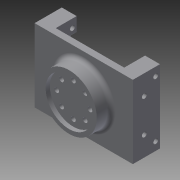
# Autodesk Inventor part: 90turnmount
Saved by Autodesk Inventor 2015 (Build 190159000, 159)
## iProperties
Created: 2016-12-16
Part Number: 90turnmount
Material: Generic
Document SubType Name: Modeling
Designer: Rudge-Top
Density: 1 g/cm^3
Appearance: Default
Author: Rudge-Top
Autodesk Inventor part; units mm, degrees
ref_plane "YZ Plane" through (0, 0, 0) normal (1, 0, 0) x (0, 1, 0)
ref_plane "XZ Plane" through (0, 0, 0) normal (0, 1, 0) x (-1, 0, 0)
ref_plane "XY Plane" through (0, 0, 0) normal (0, 0, 1) x (1, 0, 0)
sketch "Sketch1" plane through (0, 0, 0) normal (0, 1, 0) x (-1, 0, 0)
  circle A0 centre (0, 0) radius 11.25
  circle A1 centre (0, 0) radius 13.25
  dimension "d0" = 22.5
  dimension "d1" = 26.5
  constraints: 2 centre point, 2 coincident
  measures "d0" diameter of A0
  measures "d1" diameter of A1
extrude "Extrusion1" add sketch "Sketch1" along normal blind 2
sketch "Sketch2" plane through (0, 2, 0) normal (0, 1, 0) x (1, 0, 0)
  circle A0 centre (0, 0) radius 11.25 projected
  circle A1 centre (0, 0) radius 13.25 projected
extrude "Extrusion2" add sketch "Sketch2" along normal blind 5 contours A0 | A1
sketch "Sketch3" plane through (0, 7, 0) normal (0, 1, 0) x (1, 0, 0)
  line L0 (23.55, -17.5) -> (-23.55, -17.5)
  line L1 (-23.55, -17.5) -> (-23.55, 17.5)
  line L2 (-23.55, 17.5) -> (23.55, 17.5)
  line L3 (23.55, 17.5) -> (23.55, -17.5)
  point P0 (0, 0)
  dimension "d6" = 47.1
  dimension "d7" = 35
  dimension "d8" = 17.5
  dimension "d9" = 23.55
  constraints: 8 end point, 2 parallel, 1 horizontal, 1 perpendicular
  measures "d6" distance of L1.end L2.end
  measures "d7" distance of L2.end L0.start
  measures "d8" distance from line of L0 point (0, 0)
  measures "d9" distance from line of point (0, 0) L3
extrude "Extrusion3" add sketch "Sketch3" along normal blind 3
fillet "Fillet1" radius 2 1 edges at (-13.25, 7, 0)
sketch "Sketch4" plane through (0, 10, 0) normal (0, 1, 0) x (1, 0, 0)
  line L0 (-23.55, 17.5) -> (23.55, 17.5) projected
  line L1 (23.55, -17.5) -> (16.4, -17.5)
  line L2 (16.4, -17.5) -> (16.4, 17.5)
  line L3 (16.4, 17.5) -> (23.55, 17.5)
  line L4 (23.55, 17.5) -> (23.55, -17.5)
  line L5 (-23.55, -17.5) -> (-16.4, -17.5)
  line L6 (-16.4, -17.5) -> (-16.4, 17.5)
  line L7 (-16.4, 17.5) -> (-23.55, 17.5)
  line L8 (-23.55, 17.5) -> (-23.55, -17.5)
  point P0 (0, 0)
  dimension "d13" = 7.15
  dimension "d14" = 7.15
  constraints: 16 end point, 4 parallel, 2 horizontal, 2 perpendicular, 2 point on line
  measures "d13" distance of L2.end L3.end
  measures "d14" distance of L7.end L6.end
extrude "Extrusion4" add sketch "Sketch4" along normal blind 10
sketch "Sketch5" plane through (23.55, 7, 17.5) normal (1, 0, 0) x (0, 0, -1)
  line L0 (35, 0) -> (0, 0) projected
  line L1 (35, 0) -> (35, 13) projected
  line L2 (0, 13) -> (35, 13) projected
  line L3 (0, 0) -> (0, 13) projected
  line L4 (35, 13) -> (0, 13) projected
  line L5 (17.5, 13) -> (17.5, 7.9729)
  point P0 (17.5, -7)
  point P1 (25.5, 5.5)
  point P2 (31, 11)
  point P3 (9.5, 5.5)
  point P4 (4, 11)
  dimension "d17" = 5.5
  dimension "d18" = 5.5
  dimension "d19" = 8
  dimension "d20" = 13.5
  constraints: 2 end point, 2 symmetric about line, 1 midpoint, 1 vertical
  measures "d17" distance from line of L0 point (25.5, 5.5)
  measures "d18" horizontal distance of point (31, 11) point (25.5, 5.5)
  measures "d19" distance from line of L5 point (25.5, 5.5)
  measures "d20" distance from line of L5 point (31, 11)
hole "Hole1" at (23.55, 12.5, -8) at (23.55, 18, -13.5) at (23.55, 18, 13.5) at (23.55, 12.5, 8) direction (-1, 0, 0) diameter 2.3 end through all
sketch "Sketch6" plane through (0, 20, 0) normal (0, 1, 0) x (1, 0, 0)
  line L0 (23.55, -17.5) -> (23.55, 17.5) projected
  line L1 (23.55, 17.5) -> (16.4, 17.5) projected
  line L2 (16.4, 17.5) -> (16.4, -17.5) projected
  line L3 (16.4, -17.5) -> (23.55, -17.5) projected
  line L4 (16.4, 17.5) -> (16.4, -17.5) projected
  line L5 (16.4, -10.5) -> (19.3, -10.5)
  line L6 (19.3, -10.5) -> (19.3, 10.5)
  line L7 (19.3, 10.5) -> (16.4, 10.5)
  line L8 (16.4, 10.5) -> (16.4, -10.5)
  point P0 (0, 0)
  dimension "d28" = 2.9
  dimension "d29" = 21
  dimension "d30" = 7
  constraints: 8 end point, 2 parallel, 1 horizontal, 1 perpendicular, 1 point on line
  measures "d28" distance of L7.end L6.end
  measures "d29" distance of L6.end L5.end
  measures "d30" distance between parallel lines of L5 L3
extrude "Extrusion5" cut sketch "Sketch6" against normal blind 5.1 contours L2 L7 L6 L5
sketch "Sketch7" plane through (0, 20, 0) normal (0, 1, 0) x (1, 0, 0)
  line L0 (-16.4, 17.5) -> (-23.55, 17.5) projected
  line L1 (-23.55, 17.5) -> (-23.55, -17.5) projected
  line L2 (-23.55, -17.5) -> (-16.4, -17.5) projected
  line L3 (-16.4, -17.5) -> (-16.4, 17.5) projected
  line L4 (-16.4, -10.6) -> (-19.3, -10.6)
  line L5 (-19.3, -10.6) -> (-19.3, -3.6)
  line L6 (-19.3, -3.6) -> (-16.4, -3.6)
  line L7 (-16.4, -3.6) -> (-16.4, -10.6)
  line L8 (-16.4, 10.6) -> (-19.3, 10.6)
  line L9 (-19.3, 10.6) -> (-19.3, 3.6)
  line L10 (-19.3, 3.6) -> (-16.4, 3.6)
  line L11 (-16.4, 3.6) -> (-16.4, 10.6)
  point P0 (0, 0)
  dimension "d33" = 2.9
  dimension "d34" = 7
  dimension "d35" = 6.9
  dimension "d36" = 2.9
  dimension "d37" = 7
  dimension "d38" = 6.9
  constraints: 16 end point, 4 parallel, 2 horizontal, 2 perpendicular, 2 point on line
  measures "d33" distance of L5.end L6.end
  measures "d34" distance of L4.end L5.end
  measures "d35" distance between parallel lines of L2 L4
  measures "d36" distance of L10.end L9.end
  measures "d37" distance of L9.end L8.end
  measures "d38" distance between parallel lines of L0 L8
extrude "Extrusion6" cut sketch "Sketch7" against normal blind 5.1 contours L3 L10 L9 L8 | L3 L4 L5 L6
fillet "Fillet2" radius 0.5 9 edges at (-16.4, 17.45, 10.6) (-16.4, 14.9, 7.1) (-16.4, 17.45, 3.6) (-16.4, 14.9, -7.1) (-16.4, 17.45, -3.6) (-16.4, 17.45, -10.6) (16.4, 17.45, 10.5) (16.4, 14.9, 0) (16.4, 17.45, -10.5)
sketch "Sketch8" plane through (0, 2, 0) normal (0, -1, 0) x (1, 0, 0)
  point P0 (0, 0)
  point P1 (0, -8)
  point P2 (5.6569, -5.6569)
  point P3 (8, 0)
  point P4 (5.6569, 5.6569)
  point P5 (0, 8)
  point P6 (-5.6569, 5.6569)
  point P7 (-8, 0)
  point P8 (-5.6569, -5.6569)
  dimension "d42" = 8
  dimension "d45" = 360
  constraints: 9 other
  measures "d42" distance of point (0, 0) point (0, -8)
hole "Hole2" at (0, 2, -8) at (5.6569, 2, -5.6569) at (8, 2, 0) at (5.6569, 2, 5.6569) at (0, 2, 8) at (-5.6569, 2, 5.6569) at (-8, 2, 0) at (-5.6569, 2, -5.6569) direction (0, 1, 0) diameter 2.3 end through all
sketch "Sketch9" plane through (0, 10, 0) normal (0, 1, 0) x (1, 0, 0)
  line L0 (5.091, -1.9113) -> (-5.4891, -1.9113) construction
  line L1 (-5.4891, -1.9113) -> (-5.4891, 1.7202) construction
  line L2 (-5.4891, 1.7202) -> (5.091, 1.7202) construction
  line L3 (5.091, 1.7202) -> (5.091, -1.9113) construction
  line L4 (2.629, 0.3706) -> (2.629, 0.7366)
  line L5 (2.629, 0.7366) -> (3.0979, 0.7366)
  line L6 (3.0979, 0.7366) -> (3.0979, 1.6602)
  line L7 (3.0979, 1.6602) -> (3.524, 1.6602)
  line L8 (3.524, 1.6602) -> (3.524, 0.7366)
  line L9 (3.524, 0.7366) -> (5.008, 0.7366)
  line L10 (5.008, 0.7366) -> (5.008, 0.4077)
  line L11 (5.008, 0.4077) -> (3.381, -1.9113)
  line L12 (3.381, -1.9113) -> (3.0979, -1.9113)
  line L13 (3.0979, -1.9113) -> (3.0979, 0.3706)
  line L14 (3.0979, 0.3706) -> (2.629, 0.3706)
  line L15 (3.524, 0.3706) -> (3.524, -1.368)
  line L16 (3.524, -1.368) -> (4.7535, 0.3706)
  line L17 (4.7535, 0.3706) -> (3.524, 0.3706)
  line L18 (0.0211, 0.9882) -> (0.267, 1.6602)
  line L19 (0.267, 1.6602) -> (2.3316, 1.6602)
  line L20 (2.3316, 1.6602) -> (2.3316, 1.5658)
  spline S0 degree 2 poles (2.3316, 1.5658) (1.4194, 0.7337) (0.6759, -0.3186) (0.6759, -0.7561) knots 0 0 0 1 2 2 2
  spline S1 degree 2 poles (0.6759, -0.7561) (0.6759, -1.0878) (1.0848, -1.5167) (1.3679, -1.5167) knots 0 0 0 1 2 2 2
  spline S2 degree 2 poles (1.3679, -1.5167) (1.6281, -1.5167) (2.037, -1.2136) (2.1371, -0.9219) knots 0 0 0 1 2 2 2
  line L21 (2.1371, -0.9219) -> (2.2315, -0.9219)
  spline S3 degree 2 poles (2.2315, -0.9219) (2.1657, -1.3994) (1.6339, -1.9113) (1.2335, -1.9113) knots 0 0 0 1 2 2 2
  spline S4 degree 2 poles (1.2335, -1.9113) (0.8075, -1.9113) (0.2356, -1.3651) (0.2356, -0.9934) knots 0 0 0 1 2 2 2
  spline S5 degree 2 poles (0.2356, -0.9934) (0.2356, -0.7275) (0.3585, -0.4615) knots 0 0 0 1 1 1
  spline S6 degree 2 poles (0.3585, -0.4615) (0.5501, -0.0441) (0.979, 0.4249) knots 0 0 0 1 1 1
  spline S7 degree 2 poles (0.979, 0.4249) (1.6224, 1.1255) (1.7825, 1.2713) knots 0 0 0 1 1 1
  line L22 (1.7825, 1.2713) -> (0.8675, 1.2713)
  spline S8 degree 2 poles (0.8675, 1.2713) (0.5873, 1.2713) (0.3642, 1.2313) (0.1841, 1.1026) (0.1155, 0.9882) knots 0 0 0 1 2 3 3 3
  line L23 (0.1155, 0.9882) -> (0.0211, 0.9882)
  spline S9 degree 2 poles (-0.3907, -0.0698) (-0.3907, -0.6674) (-0.751, -1.531) (-1.0512, -1.7426) knots 0 0 0 1 2 2 2
  spline S10 degree 2 poles (-1.0512, -1.7426) (-1.2828, -1.9113) (-1.5316, -1.9113) knots 0 0 0 1 1 1
  spline S11 degree 2 poles (-1.5316, -1.9113) (-1.9348, -1.9113) (-2.255, -1.5024) knots 0 0 0 1 1 1
  spline S12 degree 2 poles (-2.255, -1.5024) (-2.6554, -0.9934) (-2.6554, -0.1241) knots 0 0 0 1 1 1
  spline S13 degree 2 poles (-2.6554, -0.1241) (-2.6554, 0.4849) (-2.3036, 1.3371) (-1.7603, 1.7202) (-1.5059, 1.7202) knots 0 0 0 1 2 3 3 3
  spline S14 degree 2 poles (-1.5059, 1.7202) (-1.0054, 1.7202) (-0.6709, 1.1283) knots 0 0 0 1 1 1
  spline S15 degree 2 poles (-0.6709, 1.1283) (-0.3907, 0.6308) (-0.3907, -0.0698) knots 0 0 0 1 1 1
  spline S16 degree 2 poles (-0.8968, -0.004) (-0.8968, 0.7166) (-1.0741, 1.1741) knots 0 0 0 1 1 1
  spline S17 degree 2 poles (-1.0741, 1.1741) (-1.2228, 1.5573) (-1.5144, 1.5573) knots 0 0 0 1 1 1
  spline S18 degree 2 poles (-1.5144, 1.5573) (-1.6545, 1.5573) (-1.9519, 1.3085) (-2.0291, 1.0139) knots 0 0 0 1 2 2 2
  spline S19 degree 2 poles (-2.0291, 1.0139) (-2.1492, 0.5707) (-2.1492, -0.2356) knots 0 0 0 1 1 1
  spline S20 degree 2 poles (-2.1492, -0.2356) (-2.1492, -0.8361) (-2.0263, -1.2336) knots 0 0 0 1 1 1
  spline S21 degree 2 poles (-2.0263, -1.2336) (-1.9319, -1.531) (-1.7861, -1.6539) knots 0 0 0 1 1 1
  spline S22 degree 2 poles (-1.7861, -1.6539) (-1.6803, -1.7397) (-1.5287, -1.7397) knots 0 0 0 1 1 1
  spline S23 degree 2 poles (-1.5287, -1.7397) (-1.3543, -1.7397) (-1.217, -1.5825) knots 0 0 0 1 1 1
  spline S24 degree 2 poles (-1.217, -1.5825) (-1.0312, -1.368) (-0.8968, -0.4501) (-0.8968, -0.004) knots 0 0 0 1 2 2 2
  line L24 (-5.2689, 0.9882) -> (-5.023, 1.6602)
  line L25 (-5.023, 1.6602) -> (-2.9585, 1.6602)
  line L26 (-2.9585, 1.6602) -> (-2.9585, 1.5658)
  spline S25 degree 2 poles (-2.9585, 1.5658) (-3.8706, 0.7337) (-4.6141, -0.3186) (-4.6141, -0.7561) knots 0 0 0 1 2 2 2
  spline S26 degree 2 poles (-4.6141, -0.7561) (-4.6141, -1.0878) (-4.2052, -1.5167) (-3.9221, -1.5167) knots 0 0 0 1 2 2 2
  spline S27 degree 2 poles (-3.9221, -1.5167) (-3.6619, -1.5167) (-3.253, -1.2136) (-3.1529, -0.9219) knots 0 0 0 1 2 2 2
  line L27 (-3.1529, -0.9219) -> (-3.0585, -0.9219)
  spline S28 degree 2 poles (-3.0585, -0.9219) (-3.1243, -1.3994) (-3.6562, -1.9113) (-4.0565, -1.9113) knots 0 0 0 1 2 2 2
  spline S29 degree 2 poles (-4.0565, -1.9113) (-4.4826, -1.9113) (-5.0545, -1.3651) (-5.0545, -0.9934) knots 0 0 0 1 2 2 2
  spline S30 degree 2 poles (-5.0545, -0.9934) (-5.0545, -0.7275) (-4.9315, -0.4615) knots 0 0 0 1 1 1
  spline S31 degree 2 poles (-4.9315, -0.4615) (-4.7399, -0.0441) (-4.311, 0.4249) knots 0 0 0 1 1 1
  spline S32 degree 2 poles (-4.311, 0.4249) (-3.6676, 1.1255) (-3.5075, 1.2713) knots 0 0 0 1 1 1
  line L28 (-3.5075, 1.2713) -> (-4.4225, 1.2713)
  spline S33 degree 2 poles (-4.4225, 1.2713) (-4.7027, 1.2713) (-4.9258, 1.2313) (-5.1059, 1.1026) (-5.1746, 0.9882) knots 0 0 0 1 2 3 3 3
  line L29 (-5.1746, 0.9882) -> (-5.2689, 0.9882)
  point P0 (0, 0)
  constraints: 2 other
extrude "Extrusion7" cut sketch "Sketch9" against normal blind 0.5
body "Solid1"
